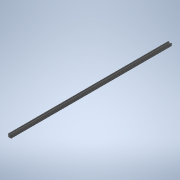
# Autodesk Inventor part: Uplotnitel-pazovyy380_-paz-6
Saved by Autodesk Inventor 2020 (Build 240168000, 168)
## iProperties
Created: 2019-04-05
Part Number: Uplotnitel-pazovyy380_-paz-6
Material: Типовые
Description: STEP AP214
Document SubType Name: Modeling
Designer: Михаил
Density: 1 g/cm^3
Appearance: По умолчанию
Sending System: SolidWorks 2018
Preprocessor: SwSTEP 2.0
Title: Z19 Óïëîòíèòåëü ïàçîâûé, ïàç 6.STEP
Author: Ïîëüçîâàòåëü Windows
Revision Number: ANY
Autodesk Inventor part; units mm, degrees
ref_plane "YZ Plane" through (0, 0, 0) normal (1, 0, 0) x (0, 1, 0)
ref_plane "XZ Plane" through (0, 0, 0) normal (0, 1, 0) x (-1, 0, 0)
ref_plane "РабПлоскость5" through (-2.9292, 0, 1000) normal (0, 0, 1) x (1, 0, 0)
sketch "Эскиз1" plane through (-2.9292, 0, 1000) normal (0, 0, 1) x (1, 0, 0)
  ellipse E0 centre (5.8827, 0.3219) end of major axis (5.857, 0.0001) minor radius 0.0779 (5.8585, 0) -> (5.958, 0.2901) ccw
  arc A0 (1.8034, 3.3833) -> (1.97, 3.9597) centre (1.8867, 3.6715) ccw
  arc A1 (3.8884, 3.9597) -> (4.0551, 3.3833) centre (3.9718, 3.6715) ccw
  line L0 (5.347, 3.757) -> (4.0551, 3.3833)
  line L1 (5.0926, 1.1901) -> (5.347, 3.757)
  ellipse E1 centre (0.8413, 1.2219) end of major axis (0.8156, 1.5437) minor radius 0.0779 (0.7659, 1.1901) -> (0.8654, 0.9) ccw
  line L2 (4.993, 0.9) -> (0.8654, 0.9)
  ellipse E2 centre (5.0172, 1.2219) end of major axis (5.0429, 1.5437) minor radius 0.0779 (4.993, 0.9) -> (5.0926, 1.1901) ccw
  line L3 (0.7659, 1.1901) -> (0.5115, 3.757)
  line L4 (1.97, 3.9597) -> (0.4478, 4.4)
  line L5 (3.8884, 3.9597) -> (5.4107, 4.4)
  line L6 (5.4107, 4.4) -> (5.5524, 5.8296)
  arc A2 (5.851, 6.1) -> (5.5524, 5.8296) centre (5.851, 5.8) ccw
  line L7 (5.851, 6.1) -> (7.0792, 6.1)
  arc A3 (7.3792, 5.8) -> (7.0792, 6.1) centre (7.0792, 5.8) ccw
  arc A4 (7.0792, 5.4) -> (7.3792, 5.7) centre (7.0792, 5.7) ccw
  line L8 (7.0792, 5.4) -> (6.4645, 5.4)
  line L9 (-0.606, 5.4) -> (-0.0995, 0.2901)
  line L10 (-1.2208, 5.4) -> (-0.606, 5.4)
  arc A5 (-1.5208, 5.7) -> (-1.2208, 5.4) centre (-1.2208, 5.7) ccw
  line L11 (-1.5208, 5.8) -> (-1.5208, 5.7)
  arc A6 (-1.2208, 6.1) -> (-1.5208, 5.8) centre (-1.2208, 5.8) ccw
  line L12 (0.0075, 6.1) -> (-1.2208, 6.1)
  arc A7 (0.3061, 5.8296) -> (0.0075, 6.1) centre (0.0075, 5.8) ccw
  line L13 (0.4478, 4.4) -> (0.3061, 5.8296)
  ellipse E3 centre (-0.0242, 0.3219) end of major axis (0.0015, 0.0001) minor radius 0.0779 (-0.0995, 0.2901) -> (0, 0) ccw
  line L14 (0, 0) -> (5.8585, 0)
  line L15 (6.4645, 5.4) -> (5.958, 0.2901)
  line L16 (7.3792, 5.8) -> (7.3792, 5.7)
  line L17 (0.5115, 3.757) -> (1.8034, 3.3833)
  point P0 (2.9292, 0)
  constraints: 36 end point, 16 point on circle, 8 centre point, 16 other
extrude "Выдавливание1" add sketch "Эскиз1" against normal blind 380
